Autodesk Inventor part; units mm, degrees
(part 6 of 6)
  line L2470 (8.9052, -43.4485) -> (9.1451, -43.4485) construction
  spline S754 degree 2 poles (9.1451, -43.4485) (9.385, -43.4485) (9.385, -43.6884) knots 0 0 0 1 1 1
  line L2471 (9.1451, -43.4485) -> (9.385, -43.4485) construction
  line L2472 (9.385, -43.4485) -> (9.385, -43.6884) construction
  spline S755 degree 2 poles (-16.3433, -61.4633) (-16.8214, -61.4633) (-17.5141, -60.7802) (-17.5141, -60.2973) knots 0 0 0 1 2 2 2
  line L2473 (-16.3433, -61.4633) -> (-16.8214, -61.4633) construction
  line L2474 (-16.8214, -61.4633) -> (-17.5141, -60.7802) construction
  line L2475 (-17.5141, -60.7802) -> (-17.5141, -60.2973) construction
  line L2476 (-17.5141, -60.2973) -> (-17.5141, -58.541)
  spline S756 degree 2 poles (-17.5141, -58.541) (-17.5141, -58.058) (-16.8214, -57.375) (-16.3433, -57.375) knots 0 0 0 1 2 2 2
  line L2477 (-17.5141, -58.541) -> (-17.5141, -58.058) construction
  line L2478 (-17.5141, -58.058) -> (-16.8214, -57.375) construction
  line L2479 (-16.8214, -57.375) -> (-16.3433, -57.375) construction
  line L2480 (-16.3433, -57.375) -> (-15.47, -57.375)
  spline S757 degree 2 poles (-15.47, -57.375) (-15.1773, -57.375) (-15.1773, -57.6677) knots 0 0 0 1 1 1
  line L2481 (-15.47, -57.375) -> (-15.1773, -57.375) construction
  line L2482 (-15.1773, -57.375) -> (-15.1773, -57.6677) construction
  spline S758 degree 2 poles (-15.1773, -57.6677) (-15.1773, -57.9604) (-15.47, -57.9604) knots 0 0 0 1 1 1
  line L2483 (-15.1773, -57.6677) -> (-15.1773, -57.9604) construction
  line L2484 (-15.1773, -57.9604) -> (-15.47, -57.9604) construction
  line L2485 (-15.47, -57.9604) -> (-16.3433, -57.9604)
  spline S759 degree 2 poles (-16.3433, -57.9604) (-16.5823, -57.9604) (-16.9287, -58.3068) (-16.9287, -58.5458) knots 0 0 0 1 2 2 2
  line L2486 (-16.3433, -57.9604) -> (-16.5823, -57.9604) construction
  line L2487 (-16.5823, -57.9604) -> (-16.9287, -58.3068) construction
  line L2488 (-16.9287, -58.3068) -> (-16.9287, -58.5458) construction
  line L2489 (-16.9287, -58.5458) -> (-16.9287, -60.2924)
  spline S760 degree 2 poles (-16.9287, -60.2924) (-16.9287, -60.5314) (-16.5823, -60.8778) (-16.3433, -60.8778) knots 0 0 0 1 2 2 2
  line L2490 (-16.9287, -60.2924) -> (-16.9287, -60.5314) construction
  line L2491 (-16.9287, -60.5314) -> (-16.5823, -60.8778) construction
  line L2492 (-16.5823, -60.8778) -> (-16.3433, -60.8778) construction
  line L2493 (-16.3433, -60.8778) -> (-15.47, -60.8778)
  spline S761 degree 2 poles (-15.47, -60.8778) (-15.1773, -60.8778) (-15.1773, -61.1705) knots 0 0 0 1 1 1
  line L2494 (-15.47, -60.8778) -> (-15.1773, -60.8778) construction
  line L2495 (-15.1773, -60.8778) -> (-15.1773, -61.1705) construction
  spline S762 degree 2 poles (-15.1773, -61.1705) (-15.1773, -61.4633) (-15.47, -61.4633) knots 0 0 0 1 1 1
  line L2496 (-15.1773, -61.1705) -> (-15.1773, -61.4633) construction
  line L2497 (-15.1773, -61.4633) -> (-15.47, -61.4633) construction
  line L2498 (-15.47, -61.4633) -> (-16.3433, -61.4633)
  spline S763 degree 2 poles (-5.566, -59.5518) (-6.0458, -59.5518) (-6.0458, -59.0719) knots 0 0 0 1 1 1
  line L2499 (-5.566, -59.5518) -> (-6.0458, -59.5518) construction
  line L2500 (-6.0458, -59.5518) -> (-6.0458, -59.0719) construction
  spline S764 degree 2 poles (-6.0458, -59.0719) (-6.0458, -58.5921) (-5.566, -58.5921) knots 0 0 0 1 1 1
  line L2501 (-6.0458, -59.0719) -> (-6.0458, -58.5921) construction
  line L2502 (-6.0458, -58.5921) -> (-5.566, -58.5921) construction
  line L2503 (-5.566, -58.5921) -> (-1.735, -58.5921)
  spline S765 degree 2 poles (-1.735, -58.5921) (-1.2632, -58.5921) (-1.2632, -59.0719) knots 0 0 0 1 1 1
  line L2504 (-1.735, -58.5921) -> (-1.2632, -58.5921) construction
  line L2505 (-1.2632, -58.5921) -> (-1.2632, -59.0719) construction
  spline S766 degree 2 poles (-1.2632, -59.0719) (-1.2632, -59.5518) (-1.735, -59.5518) knots 0 0 0 1 1 1
  line L2506 (-1.2632, -59.0719) -> (-1.2632, -59.5518) construction
  line L2507 (-1.2632, -59.5518) -> (-1.735, -59.5518) construction
  line L2508 (-1.735, -59.5518) -> (-5.566, -59.5518)
  spline S767 degree 2 poles (-20.8461, -67.4872) (-20.8461, -67.2473) (-20.6062, -67.2473) knots 0 0 0 1 1 1
  line L2509 (-20.8461, -67.4872) -> (-20.8461, -67.2473) construction
  line L2510 (-20.8461, -67.2473) -> (-20.6062, -67.2473) construction
  spline S768 degree 2 poles (-20.6062, -67.2473) (-20.3662, -67.2473) (-20.3662, -67.4872) knots 0 0 0 1 1 1
  line L2511 (-20.6062, -67.2473) -> (-20.3662, -67.2473) construction
  line L2512 (-20.3662, -67.2473) -> (-20.3662, -67.4872) construction
  line L2513 (-20.3662, -67.4872) -> (-20.3662, -70.3584)
  spline S769 degree 2 poles (-20.3662, -70.3584) (-20.3662, -70.5983) (-20.6062, -70.5983) knots 0 0 0 1 1 1
  line L2514 (-20.3662, -70.3584) -> (-20.3662, -70.5983) construction
  line L2515 (-20.3662, -70.5983) -> (-20.6062, -70.5983) construction
  spline S770 degree 2 poles (-20.6062, -70.5983) (-20.8461, -70.5983) (-20.8461, -70.3584) knots 0 0 0 1 1 1
  line L2516 (-20.6062, -70.5983) -> (-20.8461, -70.5983) construction
  line L2517 (-20.8461, -70.5983) -> (-20.8461, -70.3584) construction
  spline S771 degree 2 poles (-22.2777, -70.3584) (-22.2777, -70.5983) (-22.5176, -70.5983) knots 0 0 0 1 1 1
  line L2518 (-22.2777, -70.3584) -> (-22.2777, -70.5983) construction
  line L2519 (-22.2777, -70.5983) -> (-22.5176, -70.5983) construction
  spline S772 degree 2 poles (-22.5176, -70.5983) (-22.7576, -70.5983) (-22.7576, -70.3584) knots 0 0 0 1 1 1
  line L2520 (-22.5176, -70.5983) -> (-22.7576, -70.5983) construction
  line L2521 (-22.7576, -70.5983) -> (-22.7576, -70.3584) construction
  line L2522 (-22.7576, -70.3584) -> (-22.7576, -67.4872)
  spline S773 degree 2 poles (-22.7576, -67.4872) (-22.7576, -67.2473) (-22.5176, -67.2473) knots 0 0 0 1 1 1
  line L2523 (-22.7576, -67.4872) -> (-22.7576, -67.2473) construction
  line L2524 (-22.7576, -67.2473) -> (-22.5176, -67.2473) construction
  spline S774 degree 2 poles (-22.5176, -67.2473) (-22.2777, -67.2473) (-22.2777, -67.4872) knots 0 0 0 1 1 1
  line L2525 (-22.5176, -67.2473) -> (-22.2777, -67.2473) construction
  line L2526 (-22.2777, -67.2473) -> (-22.2777, -67.4872) construction
  spline S775 degree 2 poles (-10.553, -70.5983) (-10.7929, -70.5983) (-10.7929, -70.3584) knots 0 0 0 1 1 1
  line L2527 (-10.553, -70.5983) -> (-10.7929, -70.5983) construction
  line L2528 (-10.7929, -70.5983) -> (-10.7929, -70.3584) construction
  spline S776 degree 2 poles (-12.2405, -70.4344) (-12.2925, -70.5983) (-12.4525, -70.5983) knots 0 0 0 1 1 1
  line L2529 (-12.2405, -70.4344) -> (-12.2925, -70.5983) construction
  line L2530 (-12.2925, -70.5983) -> (-12.4525, -70.5983) construction
  spline S777 degree 2 poles (-12.4525, -70.5983) (-12.7044, -70.5983) (-12.7044, -70.3704) knots 0 0 0 1 1 1
  line L2531 (-12.4525, -70.5983) -> (-12.7044, -70.5983) construction
  line L2532 (-12.7044, -70.5983) -> (-12.7044, -70.3704) construction
  spline S778 degree 2 poles (-12.7044, -70.3704) (-12.7044, -70.3264) (-12.6884, -70.2824) knots 0 0 0 1 1 1
  line L2533 (-12.7044, -70.3704) -> (-12.7044, -70.3264) construction
  line L2534 (-12.7044, -70.3264) -> (-12.6884, -70.2824) construction
  line L2535 (-12.6884, -70.2824) -> (-11.7407, -67.4112)
  spline S779 degree 2 poles (-11.7407, -67.4112) (-11.6887, -67.2473) (-11.5167, -67.2473) knots 0 0 0 1 1 1
  line L2536 (-11.7407, -67.4112) -> (-11.6887, -67.2473) construction
  line L2537 (-11.6887, -67.2473) -> (-11.5167, -67.2473) construction
  line L2538 (-11.5167, -67.2473) -> (-10.553, -67.2473)
  spline S780 degree 2 poles (-10.553, -67.2473) (-10.3131, -67.2473) (-10.3131, -67.4872) knots 0 0 0 1 1 1
  line L2539 (-10.553, -67.2473) -> (-10.3131, -67.2473) construction
  line L2540 (-10.3131, -67.2473) -> (-10.3131, -67.4872) construction
  line L2541 (-10.3131, -67.4872) -> (-10.3131, -70.3584)
  spline S781 degree 2 poles (-10.3131, -70.3584) (-10.3131, -70.5983) (-10.553, -70.5983) knots 0 0 0 1 1 1
  line L2542 (-10.3131, -70.3584) -> (-10.3131, -70.5983) construction
  line L2543 (-10.3131, -70.5983) -> (-10.553, -70.5983) construction
  spline S782 degree 2 poles (2.1314, -67.4872) (2.1314, -67.2473) (2.3714, -67.2473) knots 0 0 0 1 1 1
  line L2544 (2.1314, -67.4872) -> (2.1314, -67.2473) construction
  line L2545 (2.1314, -67.2473) -> (2.3714, -67.2473) construction
  spline S783 degree 2 poles (2.3714, -67.2473) (2.6113, -67.2473) (2.6113, -67.4872) knots 0 0 0 1 1 1
  line L2546 (2.3714, -67.2473) -> (2.6113, -67.2473) construction
  line L2547 (2.6113, -67.2473) -> (2.6113, -67.4872) construction
  line L2548 (2.6113, -67.4872) -> (2.6113, -70.3584)
  spline S784 degree 2 poles (2.6113, -70.3584) (2.6113, -70.5983) (2.3714, -70.5983) knots 0 0 0 1 1 1
  line L2549 (2.6113, -70.3584) -> (2.6113, -70.5983) construction
  line L2550 (2.6113, -70.5983) -> (2.3714, -70.5983) construction
  spline S785 degree 2 poles (2.3714, -70.5983) (2.1314, -70.5983) (2.1314, -70.3584) knots 0 0 0 1 1 1
  line L2551 (2.3714, -70.5983) -> (2.1314, -70.5983) construction
  line L2552 (2.1314, -70.5983) -> (2.1314, -70.3584) construction
  spline S786 degree 2 poles (0.6998, -70.3584) (0.6998, -70.5983) (0.4599, -70.5983) knots 0 0 0 1 1 1
  line L2553 (0.6998, -70.3584) -> (0.6998, -70.5983) construction
  line L2554 (0.6998, -70.5983) -> (0.4599, -70.5983) construction
  spline S787 degree 2 poles (0.4599, -70.5983) (0.22, -70.5983) (0.22, -70.3584) knots 0 0 0 1 1 1
  line L2555 (0.4599, -70.5983) -> (0.22, -70.5983) construction
  line L2556 (0.22, -70.5983) -> (0.22, -70.3584) construction
  line L2557 (0.22, -70.3584) -> (0.22, -67.4872)
  spline S788 degree 2 poles (0.22, -67.4872) (0.22, -67.2473) (0.4599, -67.2473) knots 0 0 0 1 1 1
  line L2558 (0.22, -67.4872) -> (0.22, -67.2473) construction
  line L2559 (0.22, -67.2473) -> (0.4599, -67.2473) construction
  spline S789 degree 2 poles (0.4599, -67.2473) (0.6998, -67.2473) (0.6998, -67.4872) knots 0 0 0 1 1 1
  line L2560 (0.4599, -67.2473) -> (0.6998, -67.2473) construction
  line L2561 (0.6998, -67.2473) -> (0.6998, -67.4872) construction
  spline S790 degree 2 poles (11.7087, -70.1185) (11.9047, -70.1185) (12.1846, -69.8346) (12.1846, -69.6386) knots 0 0 0 1 2 2 2
  line L2562 (11.7087, -70.1185) -> (11.9047, -70.1185) construction
  line L2563 (11.9047, -70.1185) -> (12.1846, -69.8346) construction
  line L2564 (12.1846, -69.8346) -> (12.1846, -69.6386) construction
  line L2565 (12.1846, -69.6386) -> (12.1846, -68.207)
  spline S791 degree 2 poles (12.1846, -68.207) (12.1846, -68.0111) (11.9047, -67.7272) (11.7087, -67.7272) knots 0 0 0 1 2 2 2
  line L2566 (12.1846, -68.207) -> (12.1846, -68.0111) construction
  line L2567 (12.1846, -68.0111) -> (11.9047, -67.7272) construction
  line L2568 (11.9047, -67.7272) -> (11.7087, -67.7272) construction
  spline S792 degree 2 poles (10.753, -71.794) (10.753, -72.0339) (10.5131, -72.0339) knots 0 0 0 1 1 1
  line L2569 (10.753, -71.794) -> (10.753, -72.0339) construction
  line L2570 (10.753, -72.0339) -> (10.5131, -72.0339) construction
  spline S793 degree 2 poles (10.5131, -72.0339) (10.2731, -72.0339) (10.2731, -71.794) knots 0 0 0 1 1 1
  line L2571 (10.5131, -72.0339) -> (10.2731, -72.0339) construction
  line L2572 (10.2731, -72.0339) -> (10.2731, -71.794) construction
  line L2573 (10.2731, -71.794) -> (10.2731, -67.4872)
  spline S794 degree 2 poles (10.2731, -67.4872) (10.2731, -67.2473) (10.5131, -67.2473) knots 0 0 0 1 1 1
  line L2574 (10.2731, -67.4872) -> (10.2731, -67.2473) construction
  line L2575 (10.2731, -67.2473) -> (10.5131, -67.2473) construction
  line L2576 (10.5131, -67.2473) -> (11.7087, -67.2473)
  spline S795 degree 2 poles (11.7087, -67.2473) (12.1046, -67.2473) (12.6645, -67.8071) (12.6645, -68.203) knots 0 0 0 1 2 2 2
  line L2577 (11.7087, -67.2473) -> (12.1046, -67.2473) construction
  line L2578 (12.1046, -67.2473) -> (12.6645, -67.8071) construction
  line L2579 (12.6645, -67.8071) -> (12.6645, -68.203) construction
  line L2580 (12.6645, -68.203) -> (12.6645, -69.6426)
  spline S796 degree 2 poles (12.6645, -69.6426) (12.6645, -70.0385) (12.1046, -70.5983) (11.7087, -70.5983) knots 0 0 0 1 2 2 2
  line L2581 (12.6645, -69.6426) -> (12.6645, -70.0385) construction
  line L2582 (12.6645, -70.0385) -> (12.1046, -70.5983) construction
  line L2583 (12.1046, -70.5983) -> (11.7087, -70.5983) construction
  spline S797 degree 2 poles (15.0598, -70.1185) (15.2557, -70.1185) (15.5356, -69.8346) (15.5356, -69.6386) knots 0 0 0 1 2 2 2
  line L2584 (15.0598, -70.1185) -> (15.2557, -70.1185) construction
  line L2585 (15.2557, -70.1185) -> (15.5356, -69.8346) construction
  line L2586 (15.5356, -69.8346) -> (15.5356, -69.6386) construction
  spline S798 degree 2 poles (14.5799, -67.7272) (14.384, -67.7272) (14.104, -68.0111) (14.104, -68.207) knots 0 0 0 1 2 2 2
  line L2587 (14.5799, -67.7272) -> (14.384, -67.7272) construction
  line L2588 (14.384, -67.7272) -> (14.104, -68.0111) construction
  line L2589 (14.104, -68.0111) -> (14.104, -68.207) construction
  line L2590 (14.104, -68.207) -> (14.104, -69.6386)
  spline S799 degree 2 poles (14.104, -69.6386) (14.104, -69.8346) (14.384, -70.1185) (14.5799, -70.1185) knots 0 0 0 1 2 2 2
  line L2591 (14.104, -69.6386) -> (14.104, -69.8346) construction
  line L2592 (14.104, -69.8346) -> (14.384, -70.1185) construction
  line L2593 (14.384, -70.1185) -> (14.5799, -70.1185) construction
  line L2594 (14.5799, -70.1185) -> (15.0598, -70.1185)
  line L2595 (15.0598, -70.5983) -> (14.5799, -70.5983)
  spline S800 degree 2 poles (14.5799, -70.5983) (14.188, -70.5983) (13.6242, -70.0385) (13.6242, -69.6426) knots 0 0 0 1 2 2 2
  line L2596 (14.5799, -70.5983) -> (14.188, -70.5983) construction
  line L2597 (14.188, -70.5983) -> (13.6242, -70.0385) construction
  line L2598 (13.6242, -70.0385) -> (13.6242, -69.6426) construction
  line L2599 (13.6242, -69.6426) -> (13.6242, -68.203)
  spline S801 degree 2 poles (13.6242, -68.203) (13.6242, -67.8071) (14.188, -67.2473) (14.5799, -67.2473) knots 0 0 0 1 2 2 2
  line L2600 (13.6242, -68.203) -> (13.6242, -67.8071) construction
  line L2601 (13.6242, -67.8071) -> (14.188, -67.2473) construction
  line L2602 (14.188, -67.2473) -> (14.5799, -67.2473) construction
  line L2603 (14.5799, -67.2473) -> (15.7756, -67.2473)
  spline S802 degree 2 poles (15.7756, -67.2473) (16.0155, -67.2473) (16.0155, -67.4872) knots 0 0 0 1 1 1
  line L2604 (15.7756, -67.2473) -> (16.0155, -67.2473) construction
  line L2605 (16.0155, -67.2473) -> (16.0155, -67.4872) construction
  line L2606 (16.0155, -67.4872) -> (16.0155, -69.6346)
  spline S803 degree 2 poles (16.0155, -69.6346) (16.0155, -69.9945) (16.3514, -70.1385) knots 0 0 0 1 1 1
  line L2607 (16.0155, -69.6346) -> (16.0155, -69.9945) construction
  line L2608 (16.0155, -69.9945) -> (16.3514, -70.1385) construction
  spline S804 degree 2 poles (16.3514, -70.1385) (16.4994, -70.1985) (16.4994, -70.3504) knots 0 0 0 1 1 1
  line L2609 (16.3514, -70.1385) -> (16.4994, -70.1985) construction
  line L2610 (16.4994, -70.1985) -> (16.4994, -70.3504) construction
  spline S805 degree 2 poles (16.4994, -70.3504) (16.4994, -70.4504) (16.3634, -70.6023) (16.2634, -70.6023) knots 0 0 0 1 2 2 2
  line L2611 (16.4994, -70.3504) -> (16.4994, -70.4504) construction
  line L2612 (16.4994, -70.4504) -> (16.3634, -70.6023) construction
  line L2613 (16.3634, -70.6023) -> (16.2634, -70.6023) construction
  spline S806 degree 2 poles (16.2634, -70.6023) (16.2115, -70.6023) (16.1595, -70.5784) knots 0 0 0 1 1 1
  line L2614 (16.2634, -70.6023) -> (16.2115, -70.6023) construction
  line L2615 (16.2115, -70.6023) -> (16.1595, -70.5784) construction
  spline S807 degree 2 poles (16.1595, -70.5784) (15.9195, -70.4744) (15.7716, -70.2824) knots 0 0 0 1 1 1
  line L2616 (16.1595, -70.5784) -> (15.9195, -70.4744) construction
  line L2617 (15.9195, -70.4744) -> (15.7716, -70.2824) construction
  spline S808 degree 2 poles (15.7716, -70.2824) (15.4837, -70.5983) (15.0598, -70.5983) knots 0 0 0 1 1 1
  line L2618 (15.7716, -70.2824) -> (15.4837, -70.5983) construction
  line L2619 (15.4837, -70.5983) -> (15.0598, -70.5983) construction
  line L2620 (17.4551, -66.6715) -> (17.4551, -67.4152)
  spline S809 degree 2 poles (17.4551, -67.4152) (17.6431, -67.2953) (17.931, -67.0833) knots 0 0 0 1 1 1
  line L2621 (17.4551, -67.4152) -> (17.6431, -67.2953) construction
  line L2622 (17.6431, -67.2953) -> (17.931, -67.0833) construction
  spline S810 degree 2 poles (17.931, -67.0833) (18.2189, -66.8514) (18.2189, -66.6715) knots 0 0 0 1 1 1
  line L2623 (17.931, -67.0833) -> (18.2189, -66.8514) construction
  line L2624 (18.2189, -66.8514) -> (18.2189, -66.6715) construction
  spline S811 degree 2 poles (18.2189, -66.6715) (18.2189, -66.4875) (18.0989, -66.3835) knots 0 0 0 1 1 1
  line L2625 (18.2189, -66.6715) -> (18.2189, -66.4875) construction
  line L2626 (18.2189, -66.4875) -> (18.0989, -66.3835) construction
  spline S812 degree 2 poles (18.0989, -66.3835) (17.991, -66.2916) (17.839, -66.2916) knots 0 0 0 1 1 1
  line L2627 (18.0989, -66.3835) -> (17.991, -66.2916) construction
  line L2628 (17.991, -66.2916) -> (17.839, -66.2916) construction
  spline S813 degree 2 poles (17.839, -66.2916) (17.679, -66.2916) (17.5751, -66.3835) knots 0 0 0 1 1 1
  line L2629 (17.839, -66.2916) -> (17.679, -66.2916) construction
  line L2630 (17.679, -66.2916) -> (17.5751, -66.3835) construction
  spline S814 degree 2 poles (17.5751, -66.3835) (17.4551, -66.4875) (17.4551, -66.6715) knots 0 0 0 1 1 1
  line L2631 (17.5751, -66.3835) -> (17.4551, -66.4875) construction
  line L2632 (17.4551, -66.4875) -> (17.4551, -66.6715) construction
  spline S815 degree 2 poles (18.4108, -70.1185) (18.6068, -70.1185) (18.8867, -69.8346) (18.8867, -69.6386) knots 0 0 0 1 2 2 2
  line L2633 (18.4108, -70.1185) -> (18.6068, -70.1185) construction
  line L2634 (18.6068, -70.1185) -> (18.8867, -69.8346) construction
  line L2635 (18.8867, -69.8346) -> (18.8867, -69.6386) construction
  line L2636 (18.8867, -69.6386) -> (18.8867, -68.203)
  spline S816 degree 2 poles (18.8867, -68.203) (18.8867, -68.0071) (18.6068, -67.7232) (18.4108, -67.7232) knots 0 0 0 1 2 2 2
  line L2637 (18.8867, -68.203) -> (18.8867, -68.0071) construction
  line L2638 (18.8867, -68.0071) -> (18.6068, -67.7232) construction
  line L2639 (18.6068, -67.7232) -> (18.4108, -67.7232) construction
  line L2640 (18.4108, -67.7232) -> (17.931, -67.7232)
  spline S817 degree 2 poles (17.931, -67.7232) (17.735, -67.7232) (17.4551, -68.0071) (17.4551, -68.203) knots 0 0 0 1 2 2 2
  line L2641 (17.931, -67.7232) -> (17.735, -67.7232) construction
  line L2642 (17.735, -67.7232) -> (17.4551, -68.0071) construction
  line L2643 (17.4551, -68.0071) -> (17.4551, -68.203) construction
  line L2644 (17.4551, -68.203) -> (17.4551, -69.6386)
  spline S818 degree 2 poles (17.4551, -69.6386) (17.4551, -69.8346) (17.735, -70.1185) (17.931, -70.1185) knots 0 0 0 1 2 2 2
  line L2645 (17.4551, -69.6386) -> (17.4551, -69.8346) construction
  line L2646 (17.4551, -69.8346) -> (17.735, -70.1185) construction
  line L2647 (17.735, -70.1185) -> (17.931, -70.1185) construction
  line L2648 (17.931, -70.1185) -> (18.4108, -70.1185)
  spline S819 degree 2 poles (19.1306, -67.5352) (19.3666, -67.7871) (19.3666, -68.203) knots 0 0 0 1 1 1
  line L2649 (19.1306, -67.5352) -> (19.3666, -67.7871) construction
  line L2650 (19.3666, -67.7871) -> (19.3666, -68.203) construction
  line L2651 (19.3666, -68.203) -> (19.3666, -69.6426)
  spline S820 degree 2 poles (19.3666, -69.6426) (19.3666, -70.0385) (18.8067, -70.5983) (18.4108, -70.5983) knots 0 0 0 1 2 2 2
  line L2652 (19.3666, -69.6426) -> (19.3666, -70.0385) construction
  line L2653 (19.3666, -70.0385) -> (18.8067, -70.5983) construction
  line L2654 (18.8067, -70.5983) -> (18.4108, -70.5983) construction
  line L2655 (18.4108, -70.5983) -> (17.931, -70.5983)
  spline S821 degree 2 poles (17.931, -70.5983) (17.5391, -70.5983) (16.9752, -70.0385) (16.9752, -69.6426) knots 0 0 0 1 2 2 2
  line L2656 (17.931, -70.5983) -> (17.5391, -70.5983) construction
  line L2657 (17.5391, -70.5983) -> (16.9752, -70.0385) construction
  line L2658 (16.9752, -70.0385) -> (16.9752, -69.6426) construction
  line L2659 (16.9752, -69.6426) -> (16.9752, -66.6715)
  spline S822 degree 2 poles (16.9752, -66.6715) (16.9752, -66.2676) (17.2432, -66.0276) knots 0 0 0 1 1 1
  line L2660 (16.9752, -66.6715) -> (16.9752, -66.2676) construction
  line L2661 (16.9752, -66.2676) -> (17.2432, -66.0276) construction
  spline S823 degree 2 poles (17.2432, -66.0276) (17.4871, -65.8117) (17.843, -65.8117) knots 0 0 0 1 1 1
  line L2662 (17.2432, -66.0276) -> (17.4871, -65.8117) construction
  line L2663 (17.4871, -65.8117) -> (17.843, -65.8117) construction
  spline S824 degree 2 poles (17.843, -65.8117) (18.1909, -65.8117) (18.4308, -66.0236) knots 0 0 0 1 1 1
  line L2664 (17.843, -65.8117) -> (18.1909, -65.8117) construction
  line L2665 (18.1909, -65.8117) -> (18.4308, -66.0236) construction
  spline S825 degree 2 poles (18.4308, -66.0236) (18.6988, -66.2636) (18.6988, -66.6675) knots 0 0 0 1 1 1
  line L2666 (18.4308, -66.0236) -> (18.6988, -66.2636) construction
  line L2667 (18.6988, -66.2636) -> (18.6988, -66.6675) construction
  spline S826 degree 2 poles (18.6988, -66.6675) (18.6988, -67.0713) (18.4108, -67.2633) knots 0 0 0 1 1 1
  line L2668 (18.6988, -66.6675) -> (18.6988, -67.0713) construction
  line L2669 (18.6988, -67.0713) -> (18.4108, -67.2633) construction
  spline S827 degree 2 poles (18.4108, -67.2633) (18.8747, -67.2633) (19.1306, -67.5352) knots 0 0 0 1 1 1
  line L2670 (18.4108, -67.2633) -> (18.8747, -67.2633) construction
  line L2671 (18.8747, -67.2633) -> (19.1306, -67.5352) construction
  spline S828 degree 2 poles (23.9173, -70.1185) (24.1572, -70.1185) (24.1572, -70.3584) knots 0 0 0 1 1 1
  line L2672 (23.9173, -70.1185) -> (24.1572, -70.1185) construction
  line L2673 (24.1572, -70.1185) -> (24.1572, -70.3584) construction
  spline S829 degree 2 poles (24.1572, -70.3584) (24.1572, -70.5983) (23.9173, -70.5983) knots 0 0 0 1 1 1
  line L2674 (24.1572, -70.3584) -> (24.1572, -70.5983) construction
  line L2675 (24.1572, -70.5983) -> (23.9173, -70.5983) construction
  spline S830 degree 2 poles (23.9173, -70.5983) (23.6774, -70.5983) (23.6774, -70.3584) knots 0 0 0 1 1 1
  line L2676 (23.9173, -70.5983) -> (23.6774, -70.5983) construction
  line L2677 (23.6774, -70.5983) -> (23.6774, -70.3584) construction
  spline S831 degree 2 poles (23.6774, -70.3584) (23.6774, -70.1185) (23.9173, -70.1185) knots 0 0 0 1 1 1
  line L2678 (23.6774, -70.3584) -> (23.6774, -70.1185) construction
  line L2679 (23.6774, -70.1185) -> (23.9173, -70.1185) construction
  line L2680 (-23.3831, 56.0858) -> (-23.3831, 57.5254)
  circle A66 centre (21.5469, 2.4052) radius 2.6895
  circle A67 centre (14.25, 25.6049) radius 2.6895
  circle A68 centre (-14.1206, -35.4125) radius 2.6895
  circle A69 centre (20.2482, -34.283) radius 2.6895
  circle A70 centre (0.0667, -82.7708) radius 1.729
  circle A71 centre (6.7993, -78.8837) radius 1.729
  circle A72 centre (-6.6659, -86.6579) radius 1.729
  circle A73 centre (-5.2503, -28.8022) radius 2.6895
  circle A74 centre (21.5469, -7.2001) radius 2.6895
  circle A75 centre (-4.3874, -7.2001) radius 2.6895
  circle A76 centre (6.6137, 21.0639) radius 2.6895
  circle A77 centre (-14.1206, -28.8022) radius 2.6895
  circle A78 centre (20.2482, -26.9377) radius 2.6895
  circle A79 centre (-6.6659, -78.8837) radius 1.729
  circle A80 centre (6.7993, -86.6579) radius 1.729
  circle A81 centre (0.0667, -90.545) radius 1.729
  circle A82 centre (0.0667, -74.9967) radius 1.729
  circle A83 centre (-5.2503, -35.4125) radius 2.6895
  circle A84 centre (0.3144, 25.6049) radius 2.6895
  circle A85 centre (-4.3874, 2.4052) radius 2.6895
  circle A86 centre (29.7605, -100.2647) radius 1.4408
  circle A87 centre (-29.7923, -100.2647) radius 1.4408
  circle A88 centre (29.7605, 106.2491) radius 1.4408
  circle A89 centre (-29.7923, 106.2491) radius 1.4408
  circle A90 centre (3.5783, 87.9882) radius 1.5
  circle A91 centre (13.4728, 87.9882) radius 1.5
  circle A92 centre (22.7452, 87.9882) radius 1.5
  circle A93 centre (20.7295, 75.8086) radius 1.5
  circle A94 centre (9.2031, 75.8086) radius 1.5
  circle A95 centre (-0.4022, 75.8086) radius 1.5
  circle A96 centre (-10.0075, 75.8086) radius 1.5
  circle A97 centre (-19.6128, 75.8086) radius 1.5
  circle A98 centre (-19.6128, 69.0849) radius 1.5
  circle A99 centre (-10.0075, 69.0849) radius 1.5
  circle A100 centre (-0.4022, 69.0849) radius 1.5
  circle A101 centre (9.2031, 69.0849) radius 1.5
  circle A102 centre (20.7295, 69.0849) radius 1.5
  line L2681 (-24.4154, 80.9805) -> (0.0667, 80.9805)
  line L2682 (0.0667, 80.9805) -> (0.0667, 91.5512)
  line L2683 (26.1661, 86.3863) -> (26.1662, 80.5809)
  point P0 (-24.4154, 65.9583)
  dimension "d0" = 3
  dimension "d1" = 3
  dimension "d2" = 3
  dimension "d3" = 3
  dimension "d4" = 3
  dimension "d5" = 3
  dimension "d6" = 3
  dimension "d7" = 3
  dimension "d8" = 3
  dimension "d9" = 3
  dimension "d10" = 3
  dimension "d11" = 3
  dimension "d12" = 3
  constraints: 1472 end point, 128 point on circle, 103 centre point, 2 point on line, 1 horizontal, 1 perpendicular, 2496 other
  measures "d0" diameter of A95
  measures "d1" diameter of A94
  measures "d2" diameter of A93
  measures "d3" diameter of A102
  measures "d4" diameter of A101
  measures "d5" diameter of A100
  measures "d6" diameter of A96
  measures "d7" diameter of A99
  measures "d8" diameter of A97
  measures "d9" diameter of A98
  measures "d10" diameter of A90
  measures "d11" diameter of A91
  measures "d12" diameter of A92
extrude "Выдавливание1" add sketch "Эскиз1" along normal blind 3 contours L14 A9 L15 L2683 L17 A11 L18 A10 L16 L2681 L2682
sketch "Эскиз2" plane through (0, 0, 3) normal (0, 0, 1) x (1, 0, 0)
  line L0 (2.1283, 81.0852) -> (6.7676, 81.0852)
  line L1 (6.7676, 81.0852) -> (6.7676, 74.976)
  line L2 (6.7676, 74.976) -> (2.1283, 74.976)
  line L3 (2.1283, 74.976) -> (2.1283, 81.0852)
  line L4 (13.1064, 81.0852) -> (17.6997, 81.0852)
  line L5 (17.6997, 81.0852) -> (17.6997, 75.5732)
  line L6 (17.6997, 75.5732) -> (13.1064, 75.5732)
  line L7 (13.1064, 75.5732) -> (13.1064, 81.0852)
  line L8 (24.2451, 91.5512) -> (0.0667, 91.5512) projected
  line L9 (0.0667, 91.5512) -> (13.873, 91.5512)
  line L10 (13.873, 91.5512) -> (13.873, 96.2399)
  line L11 (13.873, 96.2399) -> (0.0667, 96.2399)
  line L12 (0.0667, 96.2399) -> (0.0667, 91.5512)
  point P0 (0, 0)
  constraints: 24 end point, 6 parallel, 3 horizontal, 3 perpendicular, 1 point on line
extrude "Выдавливание2" add sketch "Эскиз2" against normal blind 3 contours L8 L12 L11 L10
extrude "Выдавливание3" add sketch "Эскиз2" against normal blind 10
extrude "Выдавливание4" add sketch "Эскиз2" along normal blind 10 contours L8 L12 L11 L10
